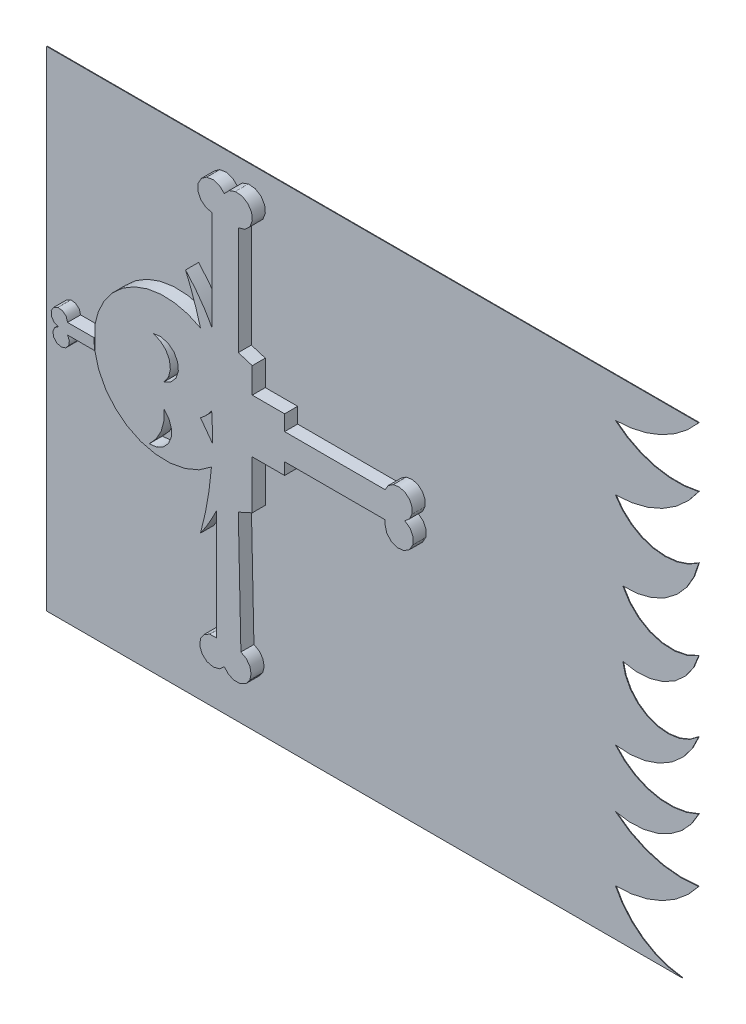
# Autodesk Inventor part: flag of ship pirate
Saved by Autodesk Inventor 2023 (Build 270158000, 158)
## iProperties
Created: 2023-10-26
Part Number: flag of ship pirate
Material: Generic
Document SubType Name: Modeling
Designer: Manaswi
Density: 1 g/cm^3
Appearance: Fine Textured - Black
Author: Manaswi
Autodesk Inventor part; units mm, degrees
ref_plane "YZ Plane" through (0, 0, 0) normal (1, 0, 0) x (0, 1, 0)
ref_plane "XZ Plane" through (0, 0, 0) normal (0, 1, 0) x (-1, 0, 0)
ref_plane "XY Plane" through (0, 0, 0) normal (0, 0, 1) x (1, 0, 0)
sketch "Sketch1" plane through (0, 0, 0) normal (0, 0, 1) x (1, 0, 0)
  point P0 (0, 0)
sketch "Sketch2" plane through (0, 0, 0) normal (0, 0, 1) x (1, 0, 0)
  line L0 (0, 0) -> (0, 750)
  line L1 (0, 750) -> (1000, 750)
  line L2 (1000, 0) -> (0, 0)
  arc A0 (872.1472, 689.3444) -> (1000, 750) centre (870.7317, 857.403) ccw
  arc A1 (872.1472, 689.3444) -> (1000, 658.5719) centre (966.1931, 799.0982) ccw
  arc A2 (872.1472, 590.6161) -> (1000, 658.5719) centre (872.5455, 744.1165) ccw
  arc A3 (872.1472, 590.6161) -> (1000, 563.6902) centre (948.1226, 634.3656) ccw
  arc A4 (883.6869, 475.2194) -> (1000, 563.6902) centre (889.4567, 588.3279) ccw
  arc A5 (883.6869, 475.2194) -> (1000, 440.6004) centre (957.0015, 508.838) ccw
  arc A6 (883.6869, 375) -> (1000, 440.6004) centre (908.84, 466.3171) ccw
  arc A7 (883.6869, 375) -> (1000, 332.8968) centre (952.2072, 382.5789) ccw
  arc A8 (872.1472, 258.53) -> (1000, 332.8968) centre (890.9368, 373.3135) ccw
  arc A9 (872.1472, 258.53) -> (1000, 230.3219) centre (953.8095, 324.8138) ccw
  arc A10 (872.1472, 170.0592) -> (1000, 230.3219) centre (899.3125, 278.1825) ccw
  arc A11 (872.1472, 170.0592) -> (1000, 134.158) centre (974.7778, 289.9436) ccw
  arc A12 (872.1472, 71.3309) -> (1000, 134.158) centre (875.3594, 226.2976) ccw
  arc A13 (872.1472, 71.3309) -> (1000, 0) centre (987.3889, 127.6425) ccw
  point P0 (974.7778, 0)
  dimension "d0" = 1000
  dimension "d1" = 750
  constraints: 28 point on circle, 14 centre point, 6 end point, 2 perpendicular, 1 vertical
  measures "d0" distance of L1.end L0.end
  measures "d1" distance of L0.start L0.end
extrude "Extrusion1" add sketch "Sketch2" along normal blind 1 contours L0 L1 A0 A1 A2 A3 A4 A5 A6 A7 A8 A9 A10 A11 A12 A13 L2
sketch "Sketch3" plane through (0, 0, 1) normal (0, 0, 1) x (1, 0, 0)
  arc A0 (255.9272, 241.4511) -> (233.0393, 579.5682) centre (37.9767, 396.5307) ccw
  arc A1 (255.9272, 241.4511) -> (233.0393, 579.5682) centre (-240.8103, 377.659) ccw
  line L0 (271.4534, 431.3865) -> (273.9174, 432.6014)
  line L1 (280.1904, 283.0201) -> (335.3049, 308.0994)
  line L2 (335.3049, 308.0994) -> (335.3049, 503.6219)
  line L3 (335.3049, 503.6219) -> (273.9174, 522.5629)
  line L4 (304.6112, 375.1252) -> (335.3049, 375.1252)
  line L5 (304.8582, 414.5966) -> (335.3049, 414.5966)
  line L6 (300.4881, 447.9105) -> (335.3049, 454.725)
  line L7 (300.4881, 345.151) -> (335.3049, 345.151)
  line L8 (335.3049, 308.0994) -> (290.4287, 308.0994)
  line L9 (335.3049, 478.7687) -> (292.5136, 478.7687)
  line L10 (398.8359, 328.3286) -> (401.8332, 328.3268)
  line L11 (401.8332, 328.3678) -> (401.8332, 328.3268)
  line L12 (335.3049, 464.4404) -> (384.9435, 464.4404)
  line L13 (384.9435, 464.4404) -> (384.9435, 464.4404)
  line L14 (384.9435, 382.5166) -> (335.3049, 382.5166)
  line L15 (384.9435, 382.5166) -> (384.9435, 464.4404)
  line L16 (273.9174, 522.5629) -> (273.9174, 676.0175)
  line L17 (313.9093, 510.2235) -> (313.9093, 676.0175)
  line L18 (280.1904, 283.0201) -> (280.1904, 114.5271)
  line L19 (313.9093, 298.3636) -> (317.8965, 114.5271)
  line L20 (384.9435, 440.7673) -> (539.0153, 440.7673)
  line L21 (384.9435, 400.7959) -> (538.9917, 400.7959)
  line L22 (538.9917, 400.7959) -> (538.9917, 394.6756)
  arc A2 (292.5136, 710.6536) -> (273.9174, 676.0175) centre (273.8735, 698.3513) ccw
  arc A3 (313.9093, 676.0175) -> (292.5136, 710.6536) centre (312.4744, 699.0575) ccw
  arc A4 (280.1904, 114.5271) -> (292.5136, 82.2759) centre (275.4611, 94.2401) ccw
  arc A5 (292.5136, 82.2759) -> (317.8965, 114.5271) centre (311.5333, 93.421) ccw
  arc A6 (569.3438, 414.5966) -> (539.0153, 440.7673) centre (559.332, 433.653) ccw
  arc A7 (538.9917, 394.6756) -> (569.3438, 414.5966) centre (560.7051, 394.6756) ccw
  arc A8 (119.3978, 413.2034) -> (119.4326, 412.4736) centre (255.9272, 419.3527) ccw
  arc A9 (408.8801, 400.7959) -> (409.9282, 414.5966) centre (255.9272, 419.3527) ccw
  arc A10 (239.4049, 572.5387) -> (236.132, 572.1502) centre (255.9272, 419.3527) ccw
  arc A11 (271.4961, 266.0669) -> (273.9174, 266.3322) centre (255.9272, 419.3527) ccw
  arc A12 (255.9272, 513.8669) -> (272.7073, 337.6534) centre (201.3368, 419.7628) ccw
  arc A13 (177.2662, 320.8702) -> (200.2183, 377.8924) centre (133.0133, 371.8129) ccw
  arc A14 (177.2662, 320.8702) -> (200.2183, 377.8924) centre (179.4288, 353.1301) ccw
  arc A15 (200.2183, 414.6034) -> (183.2381, 470.3927) centre (176.5796, 437.8874) ccw
  arc A16 (200.2183, 414.6034) -> (183.2381, 470.3927) centre (192.946, 442.8687) ccw
  line L23 (274.205, 369.9133) -> (255.9272, 394.6756)
  arc A17 (255.9272, 394.6756) -> (273.0872, 412.4459) centre (211.8011, 454.4566) ccw
  line L24 (92.5453, 419.464) -> (52.0419, 419.3528)
  line L25 (52.0419, 419.3528) -> (52.0586, 413.2472)
  line L26 (93.8919, 402.6957) -> (93.8919, 436.8299)
  arc A18 (93.8919, 402.6957) -> (52.0624, 402.6927) centre (93.8919, -288422.4778) ccw
  line L27 (52.0624, 402.6927) -> (52.0624, 402.6927)
  arc A19 (37.9745, 406.6619) -> (52.0624, 402.6927) centre (42.2022, 394.6819) ccw
  arc A20 (52.0419, 419.3528) -> (37.9745, 406.6619) centre (39.3152, 419.3178) ccw
  point P0 (0, 0)
  constraints: 54 end point, 49 point on circle, 20 centre point, 12 point on line, 6 horizontal, 5 perpendicular, 4 vertical, 2 tangent, 1 coincident, 1 parallel, 24 other
extrude "Extrusion2" add sketch "Sketch3" along normal blind 20 contours A1 A10 A0 | A12 L26 A1 A17 L23 | A0 L8 L1 | L1 L19 A5 A4 L18 | A18 A19 A20 L24 A12 | A0 L7 L2 L8 | A0 L4 L2 L7 | A0 L5 L2 L4 | A1 A0 A10 | A0 L6 L2 L5 | A0 L9 L2 L6 | L2 L12 L15 L14 | L3 L2 L9 A0 | L16 A2 A3 L17 L3 | L15 L20 A6 A7 L22 L21
body "Solid1"
